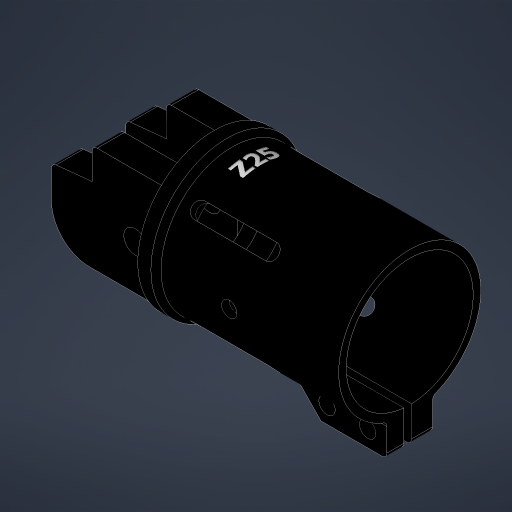
# Autodesk Inventor part: Z25_Pipe_Clamp
Saved by Autodesk Inventor 2024.1 (Build 281209000, 209)
## iProperties
Created: 2023-02-13
Part Number: Z25_Pipe_Clamp
Material: Aluminum 6061
Document SubType Name: Modeling
Designer: dzw04
Density: 2.7 g/cm^3
Appearance: Anodized - Black
Mass: 27.5691 g
Surface Area: 99.9971 cm^2
Volume: 10.2108 cm^3
Author: dzw04
Autodesk Inventor part; units mm, degrees
note: some values were not read from the file. Chosen so that the rebuilt part matches the saved one: direction of "Emboss1".
ref_plane "YZ Plane" through (0, 0, 0) normal (1, 0, 0) x (0, 1, 0)
sketch "Sketch1" plane through (0, 0, 0) normal (1, 0, 0) x (0, 1, 0)
  circle A0 centre (0, 0) radius 15
  dimension "d0" = 30
  constraints: 1 centre point, 1 coincident
  measures "d0" diameter of A0
extrude "Extrusion1" add sketch "Sketch1" along normal blind 38.6
sketch "Sketch2" plane through (38.6, 0, 0) normal (1, 0, 0) x (0, 0, -1)
  circle A0 centre (0, 0) radius 14
  circle A1 centre (0, 0) radius 15
  dimension "d3" = 28
  dimension "d4" = 30
  constraints: 2 centre point, 2 coincident
  measures "d3" diameter of A0
  measures "d4" diameter of A1
extrude "Extrusion2" cut sketch "Sketch2" against normal blind 36
chamfer "Chamfer1" distance 1 angle 45 1 edges at (2.6, 0, 14)
sketch "Sketch3" plane through (38.6, 0, 0) normal (1, 0, 0) x (0, 0, -1)
  circle A0 centre (0, 0) radius 12.5
  dimension "d10" = 25
  constraints: 1 centre point, 1 coincident
  measures "d10" diameter of A0
extrude "Extrusion3" cut sketch "Sketch3" against normal blind 36
sketch "Sketch4" plane through (2.6, 0, 0) normal (1, 0, 0) x (0, 0, -1)
  circle A0 centre (0, 0) radius 7
  dimension "d13" = 14
  constraints: 1 centre point, 1 coincident
  measures "d13" diameter of A0
extrude "Extrusion4" cut sketch "Sketch4" against normal blind 36
sketch "Sketch5" plane through (38.6, 0, 0) normal (1, 0, 0) x (0, 0, -1)
  circle A0 centre (0, 0) radius 14 projected
  line L0 (0, -14) -> (0, -19.5)
  line L1 (-4.5, -19.5) -> (4.5, -19.5)
  line L2 (4.5, -19.5) -> (4.5, -14)
  line L3 (4.5, -14) -> (-4.5, -14) construction
  line L4 (-4.5, -14) -> (-4.5, -19.5)
  line L5 (-4.5, -19.5) -> (4.5, -14) construction
  line L6 (4.5, -19.5) -> (-4.5, -14) construction
  line L7 (-4.5, -14) -> (4.5, -14) construction
  line L8 (4.5, -14) -> (4.5, -10)
  line L9 (4.5, -10) -> (-4.5, -10)
  line L10 (-4.5, -10) -> (-4.5, -14)
  circle A1 centre (0, 0) radius 12.5
  point P0 (0, -16.75)
  point P1 (4.5, -13.2571)
  point P2 (-4.5, -13.2571)
  dimension "d16" = 5.5
  dimension "d17" = 9
  dimension "d18" = 5.5
  dimension "d19" = 9
  dimension "d20" = 4
  constraints: 22 end point, 4 parallel, 3 midpoint, 2 horizontal, 2 perpendicular, 1 centre point, 1 coincident, 1 vertical, 2 other
  measures "d16" distance of L0.start L0.end
  measures "d17" distance of L3.end L2.end
  measures "d18" distance of L2.end L1.end
  measures "d19" distance of L9.end L8.end
  measures "d20" distance of L8.end L7.end
extrude "Extrusion5" add sketch "Sketch5" against normal blind 19 contours A0 L0 L1 L4 L10 | L8 L2 L1 L0 A0
fillet "Fillet1" radius 1 2 edges at (29.1, -13.2571, -4.5) (29.1, -13.2571, 4.5)
sketch "Sketch6" plane through (38.6, 0, 0) normal (1, 0, 0) x (0, 0, -1)
  line L0 (-4.5, -13.9553) -> (-4.5, -19.5) projected
  line L1 (-4.5, -19.5) -> (-1.15, -19.5)
  line L2 (-1.15, -19.5) -> (0.35, -19.5)
  line L3 (0.35, -19.5) -> (0.35, -10.5)
  line L4 (0.35, -10.5) -> (-1.15, -10.5)
  line L5 (-1.15, -10.5) -> (-1.15, -19.5)
  point P0 (0, 0)
  dimension "d27" = 3.35
  dimension "d28" = 1.5
  dimension "d29" = 9
  constraints: 10 end point, 2 horizontal, 2 parallel, 1 perpendicular
  measures "d27" distance of L0.end L1.end
  measures "d28" distance of L4.end L3.end
  measures "d29" distance of L3.end L2.end
extrude "Extrusion6" cut sketch "Sketch6" against normal blind 29
sketch "Sketch7" plane through (19.6, -19.5, 4.5) normal (0, 0, 1) x (1, 0, 0)
  circle A0 centre (15.2, 3.25) radius 1.5
  line L0 (19, 0) -> (0, 0) projected
  line L1 (19, 5.5447) -> (19, 0) projected
  circle A1 centre (7.2, 3.25) radius 1.5
  point P0 (-19.6, 19.5)
  dimension "d32" = 3
  dimension "d33" = 3.25
  dimension "d34" = 3.8
  dimension "d35" = 3
  dimension "d36" = 8
  dimension "d109" = 3.25
  constraints: 2 centre point
  measures "d32" diameter of A0
  measures "d33" distance from line of L0 A0.centre
  measures "d34" distance from line of L1 A0.centre
  measures "d35" diameter of A1
  measures "d36" distance of A0.centre A1.centre
  measures "d109" distance from line of L0 A1.centre
extrude "Extrusion7" cut sketch "Sketch7" against normal through all
sketch "Sketch8" plane through (19.6, -19.5, 4.5) normal (0, 0, 1) x (1, 0, 0)
  circle A0 centre (15.2, 3.25) radius 1.5 projected
  circle A1 centre (15.2, 3.25) radius 1.6
  circle A2 centre (7.2, 3.25) radius 1.5 projected
  circle A3 centre (7.2, 3.25) radius 1.6
  point P0 (-19.6, 19.5)
  dimension "d39" = 3.2
  dimension "d40" = 3.2
  constraints: 2 centre point, 2 coincident
  measures "d39" diameter of A1
  measures "d40" diameter of A3
extrude "Extrusion8" cut sketch "Sketch8" against normal up to surface (4.85 mm away) contours A1 | A2 | A3
fillet "Fillet2" radius 1 2 edges at (38.6, -19.5, 2.825) (38.6, -19.5, -2.425)
sketch "Sketch10" plane through (19.6, -13.9553, 4.5) normal (0, 0, 1) x (1, 0, 0)
  circle A0 centre (15.2, -2.2947) radius 1.6 projected
  circle A1 centre (15.2, -2.2947) radius 2.875
  circle A2 centre (7.2, -2.2947) radius 1.6 projected
  circle A3 centre (7.2, -2.2947) radius 2.875
  point P0 (-19.6, 13.9553)
  dimension "d48" = 5.75
  dimension "d49" = 5.75
  constraints: 2 centre point, 2 coincident
  measures "d48" diameter of A1
  measures "d49" diameter of A3
extrude "Extrusion10" cut sketch "Sketch10" along normal blind 19
ref_plane "Work Plane1" through (19.6, -19.5, 0) normal (0, 0, 1) x (1, 0, 0)
sketch "Sketch11" plane through (19.6, -19.5, 0) normal (0, 0, 1) x (1, 0, 0)
  line L0 (0, 0) -> (0, 5.5447) construction
  line L1 (0, 0) -> (0, 23.1484) construction
  line L2 (0, 19.5) -> (0, 5.5)
  line L3 (0, 5.5) -> (0, -4.5)
  line L4 (0, -4.5) -> (10, -4.5)
  line L5 (10, -4.5) -> (0, 5.5)
  line L6 (0, 19.5) -> (-19.6, 19.5)
  line L7 (26.72, 19.5) -> (-27.32, 19.5) projected
  dimension "d52" = 14
  dimension "d53" = 10
  dimension "d54" = 10
  constraints: 12 end point, 3 point on line, 1 horizontal, 1 perpendicular, 1 vertical
  measures "d52" distance of L2.start L2.end
  measures "d53" distance of L2.end L3.end
  measures "d54" distance of L3.end L4.end
revolve "Revolution1" cut sketch "Sketch11" angle 360 about axis through (38.6, 0, 0) along (-1, 0, 0)
sketch "Sketch12" plane through (0, 0, 0) normal (-1, 0, 0) x (0, 0, 1)
  line L0 (-4.625, -10.5) -> (4.625, -10.5)
  line L1 (4.625, -10.5) -> (4.625, 10.5)
  line L2 (4.625, 10.5) -> (-4.625, 10.5)
  line L3 (-4.625, 10.5) -> (-4.625, -10.5)
  circle A0 centre (0, 0) radius 7 projected
  line L4 (-4.625, -10.5) -> (4.625, 10.5) construction
  line L5 (4.625, -10.5) -> (-4.625, 10.5) construction
  line L6 (4.625, -10.5) -> (10, -10.5)
  line L7 (10, -10.5) -> (10, 10.5)
  line L8 (10, 10.5) -> (4.625, 10.5)
  line L9 (4.625, 10.5) -> (4.625, -10.5)
  line L10 (-4.625, -10.5) -> (-10, -10.5)
  line L11 (-10, -10.5) -> (-10, 10.5)
  line L12 (-10, 10.5) -> (-4.625, 10.5)
  line L13 (-4.625, 10.5) -> (-4.625, -10.5)
  dimension "d56" = 9.25
  dimension "d57" = 21
  dimension "d58" = 5.375
  dimension "d59" = 5.375
  dimension "d60" = 21
  constraints: 28 end point, 6 parallel, 3 horizontal, 3 perpendicular, 2 midpoint, 1 point on line
  measures "d56" distance of L2.end L1.end
  measures "d57" distance of L1.end L0.end
  measures "d58" distance of L8.end L7.end
  measures "d59" distance between parallel lines of L3 L11
  measures "d60" distance between parallel lines of L10 L12
extrude "Extrusion11" add sketch "Sketch12" along normal blind 22 contours L10 L11 L12 L3 A0 | L1 A0 L8 L7 L6 | A0 L3 | L1 A0
sketch "Sketch13" plane through (0, -10.5, 10) normal (0, 0, 1) x (1, 0, 0)
  circle A0 centre (-5.5, 8.75) radius 2.25
  line L0 (0, -4.5) -> (0, 25.5) projected
  line L1 (0, 0) -> (-22, 0) projected
  point P0 (0, 10.5)
  dimension "d63" = 5.5
  dimension "d64" = 8.75
  dimension "d67" = 4.5
  constraints: 1 centre point
  measures "d63" distance from line of L0 A0.centre
  measures "d64" distance from line of L1 A0.centre
  measures "d67" diameter of A0
extrude "Extrusion12" cut sketch "Sketch13" against normal through all
sketch "Sketch14" plane through (0, -10.5, 10) normal (0, 0, 1) x (1, 0, 0)
  line L0 (0, 21) -> (-22, 21) projected
  line L1 (0, 21) -> (-14, 21)
  line L2 (-14, 21) -> (-14, 14.8)
  line L3 (-22, 21) -> (-22, 0) projected
  line L4 (-22, 0) -> (-22, 14)
  line L5 (-22, 14) -> (-14, 14.8)
  line L6 (-22, 14) -> (-22, 21)
  line L7 (-22, 21) -> (-14, 21)
  point P0 (0, 10.5)
  dimension "d68" = 14
  dimension "d69" = 6.2
  dimension "d70" = 14
  constraints: 12 end point, 2 perpendicular, 2 point on line, 1 collinear
  measures "d68" distance of L0.start L1.end
  measures "d69" distance of L1.end L2.end
  measures "d70" distance of L3.end L4.end
extrude "Extrusion13" cut sketch "Sketch14" against normal through all
fillet "Fillet3" radius 7.5 2 edges at (-22, -10.5, -7.3125) (-22, -10.5, 7.3125)
fillet "Fillet4" radius 1 4 edges at (-22, 3.5, -7.3125) (-22, 3.5, 7.3125) (-14, 10.5, 7.3125) (-14, 10.5, -7.3125)
sketch "Sketch15" plane through (0, -10.5, -10) normal (0, 0, -1) x (-1, 0, 0)
  circle A0 centre (14, 8.75) radius 1.5
  circle A1 centre (5.5, 17.5) radius 1.5
  circle A2 centre (5.5, 8.75) radius 2.25 projected
  arc A3 (14, 20) -> (13, 21) centre (13, 20) ccw projected
  line L0 (0, 21) -> (13, 21) projected
  line L1 (0, 0) -> (0, 21) projected
  line L2 (0, 0) -> (14.5, 0) projected
  arc A4 (14.5, 0) -> (22, 7.5) centre (14.5, 7.5) ccw projected
  line L3 (22, 13.095) -> (22, 7.5) projected
  arc A5 (22, 13.095) -> (21.0995, 14.09) centre (21, 13.095) ccw projected
  line L4 (21.0995, 14.09) -> (14, 14.8) projected
  line L5 (14, 14.8) -> (14, 20) projected
  point P0 (0, 10.5)
  dimension "d75" = 3
  dimension "d76" = 3
  dimension "d77" = 14
  dimension "d78" = 3.5
  dimension "d79" = 5.5
  constraints: 2 centre point, 1 horizontal alignment
  measures "d75" diameter of A1
  measures "d76" diameter of A0
  measures "d77" distance from line of L1 A0.centre
  measures "d78" distance from line of L0 A1.centre
  measures "d79" distance from line of L1 A1.centre
extrude "Extrusion14" cut sketch "Sketch15" against normal up to surface (5.375 mm away) contours A0 | A1
sketch "Sketch16" plane through (19.6, -19.5, 0) normal (0, 0, 1) x (1, 0, 0)
  line L0 (-19.6, 4.5) -> (-19.6, 34.5) projected
  line L1 (-19.6, 19.5) -> (-36.6, 19.5)
  line L2 (-19.6, 14.2455) -> (-19.6, 24.7545) projected
  line L3 (-19.6, 19.5) -> (-2.6, 19.5)
  circle A0 centre (-2.6, 19.5) radius 1.5
  dimension "d82" = 17
  dimension "d83" = 17
  dimension "d84" = 3
  constraints: 4 end point, 2 perpendicular, 1 centre point, 1 coincident
  measures "d82" distance of L1.start L1.end
  measures "d83" distance of L1.start L3.end
  measures "d84" diameter of A0
extrude "Extrusion15" cut sketch "Sketch16" along normal through all both and the other way through all
ref_plane "Work Plane2" through (38.6, 0, 0) normal (0, 0.7071068, 0.7071068) x (-1, 0, 0)
sketch "Sketch17" plane through (38.6, 0, 0) normal (0, 0.7071068, 0.7071068) x (-1, 0, 0)
  line L0 (19, 5.5802) -> (19, 9.6489) projected
  line L1 (19, 9.6489) -> (29, 9.6489) projected
  line L2 (29, 9.6489) -> (29, 10.6792) projected
  line L3 (29, 10.6792) -> (19, 10.6792) projected
  line L4 (19, 10.6792) -> (19, 12.8398) projected
  line L5 (0, 12.8398) -> (19, 12.8398) projected
  line L6 (0, 5.5802) -> (0, 12.8398) projected
  line L7 (19, 5.5802) -> (0, 5.5802) projected
  line L8 (35, -14) -> (35, 14) projected
  line L9 (38.6, 15) -> (38.6, -15) projected
  line L10 (0, -12.5) -> (0, 12.5) projected
  line L11 (0, 0) -> (17.5, 0)
  line L12 (17.5, 0) -> (31.5, 0)
  line L13 (17.5, 0) -> (31.5, 0) construction
  line L14 (17.5, -1.5) -> (31.5, -1.5)
  line L15 (31.5, 1.5) -> (17.5, 1.5)
  arc A0 (17.5, 1.5) -> (17.5, -1.5) centre (17.5, 0) ccw
  arc A1 (31.5, -1.5) -> (31.5, 1.5) centre (31.5, 0) ccw
  point P0 (38.6, 0)
  point P1 (0, 9.6145)
  point P2 (0, 8.5879)
  point P3 (24.5, 0)
  dimension "d88" = 17.5
  dimension "d89" = 14
  dimension "d90" = 3
  constraints: 12 end point, 4 point on circle, 4 tangent, 2 centre point, 2 horizontal, 2 midpoint, 1 parallel, 1 point on line, 2 other
  measures "d88" distance of L11.start L11.end
  measures "d89" distance of L11.end L12.end
  measures "d90" diameter of A1
extrude "Extrusion16" cut sketch "Sketch17" against normal through all contours A0 L15 A1 L14
pattern_circular "Circular Pattern1" count 4 over 360 about axis through (38.6, 0, 0) along (-1, 0, 0) of "Extrusion16"
ref_plane "Work Plane3" through (0, 14, 0) normal (0, 1, 0) x (-1, 0, 0)
sketch "Sketch18" plane through (0, 14, 0) normal (0, 1, 0) x (-1, 0, 0)
  line L0 (-6.3441, 3.806) -> (-6.3441, -4.1477) construction
  line L1 (-6.3441, -4.1477) -> (-9.5177, -4.1477) construction
  line L2 (-9.5177, -4.1477) -> (-9.5177, 3.806) construction
  line L3 (-9.5177, 3.806) -> (-6.3441, 3.806) construction
  line L4 (-9.4534, 1.2775) -> (-9.4534, 3.6948)
  line L5 (-9.4534, 3.6948) -> (-8.8825, 3.6948)
  line L6 (-8.8825, 3.6948) -> (-6.9843, 2.2884)
  line L7 (-6.9843, 2.2884) -> (-6.9843, 3.6207)
  line L8 (-6.9843, 3.6207) -> (-6.4034, 3.6207)
  line L9 (-6.4034, 3.6207) -> (-6.4034, 1.3591)
  line L10 (-6.4034, 1.3591) -> (-6.9843, 1.3591)
  line L11 (-6.9843, 1.3591) -> (-8.8726, 2.7605)
  line L12 (-8.8726, 2.7605) -> (-8.8726, 1.2775)
  line L13 (-8.8726, 1.2775) -> (-9.4534, 1.2775)
  line L14 (-9.4534, -1.3548) -> (-9.4534, 0.887)
  line L15 (-9.4534, 0.887) -> (-8.9566, 0.887)
  spline S0 degree 2 poles (-8.9566, 0.887) (-8.7292, 0.6028) (-8.3288, 0.148) (-8.1484, -0.0225) knots 0 0 0 1 2 2 2
  spline S1 degree 2 poles (-8.1484, -0.0225) (-7.9136, -0.2475) (-7.5552, -0.4477) (-7.3674, -0.4477) knots 0 0 0 1 2 2 2
  spline S2 degree 2 poles (-7.3674, -0.4477) (-7.1548, -0.4477) (-6.9274, -0.1931) (-6.9274, 0.0343) knots 0 0 0 1 2 2 2
  spline S3 degree 2 poles (-6.9274, 0.0343) (-6.9274, 0.1505) (-6.9843, 0.3581) (-7.0287, 0.4644) knots 0 0 0 1 2 2 2
  spline S4 degree 2 poles (-7.0287, 0.4644) (-7.0757, 0.5682) (-7.1746, 0.7165) (-7.1993, 0.7536) knots 0 0 0 1 2 2 2
  line L16 (-7.1993, 0.7536) -> (-7.1993, 0.8129)
  line L17 (-7.1993, 0.8129) -> (-6.5344, 0.8129)
  spline S5 degree 2 poles (-6.5344, 0.8129) (-6.4726, 0.6843) (-6.3441, 0.1356) (-6.3441, -0.1189) knots 0 0 0 1 2 2 2
  spline S6 degree 2 poles (-6.3441, -0.1189) (-6.3441, -0.6627) (-6.8285, -1.2213) (-7.266, -1.2213) knots 0 0 0 1 2 2 2
  spline S7 degree 2 poles (-7.266, -1.2213) (-7.5354, -1.2213) (-8.0545, -0.9667) (-8.3511, -0.6726) knots 0 0 0 1 2 2 2
  spline S8 degree 2 poles (-8.3511, -0.6726) (-8.534, -0.4872) (-8.8182, -0.1387) (-8.8775, -0.0621) knots 0 0 0 1 2 2 2
  line L18 (-8.8775, -0.0621) -> (-8.8775, -1.3548)
  line L19 (-8.8775, -1.3548) -> (-9.4534, -1.3548)
  spline S9 degree 2 poles (-8.4203, -3.9574) (-8.66, -3.9574) (-9.0654, -3.7943) (-9.2112, -3.6336) knots 0 0 0 1 2 2 2
  spline S10 degree 2 poles (-9.2112, -3.6336) (-9.357, -3.4729) (-9.5177, -3.033) (-9.5177, -2.7117) knots 0 0 0 1 2 2 2
  spline S11 degree 2 poles (-9.5177, -2.7117) (-9.5152, -2.3706) (-9.404, -1.8812) (-9.3323, -1.7206) knots 0 0 0 1 2 2 2
  line L20 (-9.3323, -1.7206) -> (-8.6674, -1.7206)
  line L21 (-8.6674, -1.7206) -> (-8.6674, -1.7898)
  spline S12 degree 2 poles (-8.6674, -1.7898) (-8.6996, -1.8491) (-8.7836, -1.9924) (-8.8281, -2.1086) knots 0 0 0 1 2 2 2
  spline S13 degree 2 poles (-8.8281, -2.1086) (-8.8701, -2.2174) (-8.927, -2.4423) (-8.927, -2.5782) knots 0 0 0 1 2 2 2
  spline S14 degree 2 poles (-8.927, -2.5782) (-8.927, -2.6969) (-8.8676, -2.9737) (-8.7886, -3.0577) knots 0 0 0 1 2 2 2
  spline S15 degree 2 poles (-8.7886, -3.0577) (-8.7268, -3.1195) (-8.576, -3.1887) (-8.4499, -3.1887) knots 0 0 0 1 2 2 2
  spline S16 degree 2 poles (-8.4499, -3.1887) (-8.3412, -3.1887) (-8.1879, -3.0997) (-8.141, -3.0281) knots 0 0 0 1 2 2 2
  spline S17 degree 2 poles (-8.141, -3.0281) (-8.0718, -2.9242) (-8.0322, -2.6276) (-8.0322, -2.5214) knots 0 0 0 1 2 2 2
  spline S18 degree 2 poles (-8.0322, -2.5214) (-8.0322, -2.3533) (-8.0866, -2.0345) (-8.1163, -1.9183) knots 0 0 0 1 2 2 2
  line L22 (-8.1163, -1.9183) -> (-8.1163, -1.8516)
  line L23 (-8.1163, -1.8516) -> (-6.4034, -1.8516)
  line L24 (-6.4034, -1.8516) -> (-6.4034, -3.8734)
  line L25 (-6.4034, -3.8734) -> (-6.9793, -3.8734)
  line L26 (-6.9793, -3.8734) -> (-6.9793, -2.5757)
  line L27 (-6.9793, -2.5757) -> (-7.486, -2.5757)
  spline S19 degree 2 poles (-7.486, -2.5757) (-7.4811, -2.6375) (-7.4761, -2.8081) (-7.4761, -2.855) knots 0 0 0 1 2 2 2
  spline S20 degree 2 poles (-7.4761, -2.855) (-7.4761, -3.075) (-7.5651, -3.4458) (-7.6565, -3.5916) knots 0 0 0 1 2 2 2
  spline S21 degree 2 poles (-7.6565, -3.5916) (-7.7702, -3.7646) (-8.1484, -3.9574) (-8.4203, -3.9574) knots 0 0 0 1 2 2 2
  point P0 (0, 0)
  dimension "d0" = 30
  constraints: 2 other
emboss "Emboss1" sketch "Sketch18" operation cut depth 0.1 direction (0, -1, 0)
thread "Thread4" size "M3x0.5" class "6H" standard "ANSI Metric M Profile" full length
thread "Thread5" size "M3x0.5" class "6H" standard "ANSI Metric M Profile" full length
thread "Thread6" size "M3x0.5" class "6H" standard "ANSI Metric M Profile" full length
thread "Thread7" size "M3x0.5" class "6H" standard "ANSI Metric M Profile" full length
equation "\"d35\" = d32"
equation "\"d109\" = d33"
equation "\"d59\" = d58"
equation "\"d60\" = d57"
equation "\"d76\" = d75"
equation "\"d80\" = d76"
body "Solid1"
